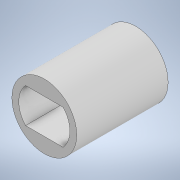
# Autodesk Inventor part: Motor Fäste-Test
Saved by Autodesk Inventor 2021 (Build 250183000, 183)
## iProperties
Created: 2024-12-11
Part Number: Motor Fäste-Test
Material: Generic
Document SubType Name: Modeling
Designer: 24lucsil
Density: 1 g/cm^3
Appearance: Default
Author: 24lucsil
Autodesk Inventor part; units mm, degrees
ref_plane "YZ Plane" through (0, 0, 0) normal (1, 0, 0) x (0, 1, 0)
ref_plane "XZ Plane" through (0, 0, 0) normal (0, 1, 0) x (-1, 0, 0)
ref_plane "XY Plane" through (0, 0, 0) normal (0, 0, 1) x (1, 0, 0)
sketch "Sketch1" plane through (0, 0, 0) normal (0, 0, 1) x (1, 0, 0)
  circle A0 centre (0, 0) radius 2.8
  line L0 (0, 2.8) -> (0, 1.9)
  line L1 (0, -2.8) -> (0, -1.9)
  line L2 (-2.0567, -1.9) -> (2.0567, -1.9)
  line L3 (2.0567, 1.9) -> (-2.0567, 1.9)
  circle A1 centre (0, 0) radius 3.55
  dimension "d0" = 5.6
  dimension "d1" = 0.9
  dimension "d2" = 0.9
  dimension "d3" = 4.1134
  dimension "d4" = 4.1134
  dimension "d5" = 7.1
  constraints: 8 end point, 6 point on circle, 2 centre point, 2 coincident, 2 horizontal, 2 vertical
  measures "d0" diameter of A0
  measures "d1" distance of L0.start L0.end
  measures "d2" distance of L1.start L1.end
  measures "d3" distance of L3.start L3.end
  measures "d4" distance of L2.start L2.end
  measures "d5" diameter of A1
extrude "Extrusion1" add sketch "Sketch1" along normal blind 10 contours L3 L0 A0 | A0 L1 L2 | L0 L3 A0 | A0 L2 L1 | A1
body "Solid1"
